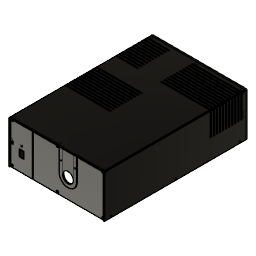
Alt Case (metal) 10mm (Autodesk Fusion 360 design; units mm, degrees)
Autodesk Fusion 360 part; units mm, degrees
sketch "Front" plane through (0, -75, 0) normal (0, -1, 0) x (1, 0, 0)
  line L0 (105, 0) -> (-170, 0)
  line L1 (-170, 0) -> (-170, -10)
  line L2 (-170, -10) -> (107, -10)
  line L3 (-170, 115) -> (105, 115)
  line L4 (-170, 115) -> (-170, 0)
  line L5 (-170, 0) -> (-170, -10)
  line L6 (105, 115) -> (105, 0)
  line L7 (-172, 117) -> (-172, -10)
  line L8 (-172, 117) -> (107, 117)
  line L9 (107, 117) -> (107, -10)
  line L10 (-170, -10) -> (-172, -10)
  circle A0 centre (0, 48) radius 12.5 construction
  line L11 (-104.1, 115) -> (-104.1, -10)
  line L12 (-105.9, 115) -> (-105.9, -10)
  line L13 (-105.9, -10) -> (-104.1, -10)
  line L14 (-144.45, 48) -> (-131.45, 48)
  line L15 (-131.45, 48) -> (-131.45, 28)
  line L16 (-131.45, 28) -> (-144.45, 28)
  line L17 (-144.45, 28) -> (-144.45, 48)
  line L18 (-131.45, 38) -> (-105.9, 38) construction
  line L19 (-144.45, 38) -> (-170, 38) construction
  circle A1 centre (-137.95, 58) radius 1.6
  circle A2 centre (-137.95, 58) radius 3.5
  line L20 (-108, 115) -> (-102, 115)
  line L21 (-102, 115) -> (-102, -10)
  line L22 (-102, -10) -> (-108, -10)
  line L23 (-108, -10) -> (-108, 115)
  line L24 (-105, 115) -> (-105, 111.6183) construction
  line L25 (-105.9, 104.1973) -> (-104.1, 104.1973) construction
  line L26 (-105, 115) -> (-105, -10)
  line L27 (-102, 106) -> (-108, 106)
  line L28 (-15.3704, -10) -> (15.3704, -10)
  line L29 (-12.8704, 115) -> (-17.8704, 115)
  line L30 (105, 115) -> (97, 115)
  line L31 (97, 115) -> (97, 107)
  line L32 (97, 107) -> (105, 107)
  line L33 (105, 107) -> (105, 115)
  line L34 (105, 115) -> (97, 107) construction
  line L35 (97, 115) -> (105, 107) construction
  line L36 (-36.5, 115) -> (-28.5, 115)
  line L37 (-28.5, 115) -> (-28.5, 107)
  line L38 (-28.5, 107) -> (-36.5, 107)
  line L39 (-36.5, 107) -> (-36.5, 115)
  line L40 (-36.5, 115) -> (-28.5, 107) construction
  line L41 (-28.5, 115) -> (-36.5, 107) construction
  line L42 (-170, 115) -> (-162, 115)
  line L43 (-162, 115) -> (-162, 107)
  line L44 (-162, 107) -> (-170, 107)
  line L45 (-170, 107) -> (-170, 115)
  line L46 (-170, 115) -> (-162, 107) construction
  line L47 (-162, 115) -> (-170, 107) construction
  line L48 (105, 57.5) -> (97, 57.5)
  line L49 (97, 57.5) -> (97, 49.5)
  line L50 (97, 49.5) -> (105, 49.5)
  line L51 (105, 49.5) -> (105, 57.5)
  line L52 (105, 57.5) -> (97, 49.5) construction
  line L53 (97, 57.5) -> (105, 49.5) construction
  line L54 (-170, 57.5) -> (-162, 57.5)
  line L55 (-162, 57.5) -> (-162, 49.5)
  line L56 (-162, 49.5) -> (-170, 49.5)
  line L57 (-170, 49.5) -> (-170, 57.5)
  line L58 (-170, 57.5) -> (-162, 49.5) construction
  line L59 (-162, 57.5) -> (-170, 49.5) construction
  line L60 (-200, 53.5) -> (146.6101, 53.5) construction
  circle A3 centre (-32.5, 111) radius 1.45
  circle A4 centre (101, 111) radius 1.45
  circle A5 centre (101, 53.5) radius 1.45
  circle A6 centre (-166, 111) radius 1.45
  circle A7 centre (-166, 53.5) radius 1.45
  line L61 (-28.5, 107) -> (-20.5, 115)
  line L62 (-28.5, 107) -> (-32.5, 107) construction
  line L63 (-85.5, -10) -> (-124.5, -10)
  line L64 (-124.5, -10) -> (-124.5, 20)
  line L65 (-124.5, 20) -> (-85.5, 20)
  line L66 (-85.5, 20) -> (-85.5, -10)
  line L67 (-85.5, -10) -> (-124.5, 20) construction
  line L68 (-124.5, -10) -> (-85.5, 20) construction
  line L69 (61.5, -10) -> (22.5, -10)
  line L70 (22.5, -10) -> (22.5, 20)
  line L71 (22.5, 20) -> (61.5, 20)
  line L72 (61.5, 20) -> (61.5, -10)
  line L73 (61.5, -10) -> (22.5, 20) construction
  line L74 (22.5, -10) -> (61.5, 20) construction
  line L75 (97, 57.5) -> (105, 65.5)
  line L76 (97, 57.5) -> (106.5359, 57.5) construction
  line L77 (105, 0) -> (105, -10)
  line L78 (15.5, 48) -> (15.5, 115)
  line L79 (-15.5, 115) -> (-15.5, 48)
  line L80 (-162, 57.5) -> (-170, 65.5)
  line L81 (-162, 57.5) -> (-152.8212, 57.5) construction
  line L82 (12.5, 0) -> (2.5, 0)
  line L83 (2.5, 0) -> (2.5, 5)
  line L84 (2.5, 5) -> (12.5, 5)
  line L85 (12.5, 5) -> (12.5, 0)
  line L86 (-155, 0) -> (-145, 0)
  line L87 (-145, 0) -> (-145, 5)
  line L88 (-145, 5) -> (-155, 5)
  line L89 (-155, 5) -> (-155, 0)
  circle A8 centre (-166, -5) radius 1.75
  circle A9 centre (-32.5, -5) radius 1.75
  circle A10 centre (101, -5) radius 1.75
  arc A11 (-15.5, 48) -> (15.5, 48) centre (0, 48) ccw
  line L90 (-25.5, 115) -> (-25.5, 48)
  arc A12 (-25.5, 48) -> (25.5, 48) centre (0, 48) ccw
  line L91 (25.5, 48) -> (25.5, 115)
  circle A13 centre (0, 48) radius 15.5
  circle A14 centre (20.5, 81.5) radius 1.75
  circle A15 centre (-20.5, 81.5) radius 1.75
  line L92 (-25.5, 81.5) -> (-15.5, 81.5) construction
  line L93 (15.5, 81.5) -> (25.5, 81.5) construction
  line L94 (0, 48) -> (0, 115) construction
  point P0 (-137.95, 48)
  point P1 (-105, 104.1973)
  point P2 (101, 111)
  point P3 (-32.5, 111)
  point P4 (-166, 111)
  point P5 (101, 53.5)
  point P6 (-166, 53.5)
  point P7 (-105, 5)
  point P8 (42, 5)
  point P9 (-32.5, 117)
  point P10 (0, 81.5)
  dimension "d597" = 2
  dimension "d607" = 115
  dimension "d617" = 105
  dimension "d623" = 1.8
  dimension "d625" = 13
  dimension "d626" = 20
  dimension "d628" = 3.2
  dimension "d629" = 7
  dimension "d630" = 10
  dimension "d634" = 6
  dimension "d639" = 9
  dimension "d806" = 8
  dimension "d808" = 2.9
  dimension "d812" = 45
  dimension "d841" = 39
  dimension "d842" = 30
  dimension "d846" = 65
  dimension "d847" = 65
  dimension "d870" = 45
  dimension "d1" = 275
  dimension "d2" = 48
  dimension "d3" = 25
  dimension "d4" = 31
  dimension "d6" = 53.5
  dimension "d24" = 10
  dimension "d30" = 135
  dimension "d49" = 10
  dimension "d50" = 5
  dimension "d51" = 10
  dimension "d52" = 15
  dimension "d95" = 3.5
  dimension "d97" = 5
  dimension "d100" = 267
  dimension "d101" = 0
  dimension "d102" = 10
  dimension "d103" = 3.5
  dimension "d111" = 4
  constraint horizontal L3
  constraint coincident L0.end L1.start
  constraint coincident L1.end L2.start
  constraint coincident L0.start L6.end
  constraint coincident L3 L11.start
  constraint coincident L2 L11.end
  constraint perpendicular L2 L11
  constraint perpendicular L11 L13
  constraint horizontal L14
  constraint vertical L15
  constraint horizontal L16
  constraint vertical L17
  constraint midpoint L15 L18.start
  constraint coincident L12 L18.end
  constraint perpendicular L12 L18
  constraint midpoint L17 L19.start
  constraint coincident L4 L19.end
  constraint perpendicular L17 L19
  constraint equal L18 L19
  constraint concentric A1 A2
  constraint midpoint L14 P0
  constraint vertical A1.centre P0
  constraint horizontal L20
  constraint vertical L21
  constraint horizontal L22
  constraint vertical L23
  constraint coincident L2 L21.end
  constraint midpoint L20 L24.start
  constraint perpendicular L20 L24
  constraint coincident L12 L25.start
  constraint coincident L11 L25.end
  constraint perpendicular L11 L25
  constraint midpoint L25 P1
  constraint vertical L24.end P1
  constraint coincident L3 L20.start
  constraint midpoint L22 L26.end
  constraint coincident L21 L27.start
  constraint coincident L23 L27.end
  constraint perpendicular L23 L27
  constraint horizontal A0.centre P0
  constraint coincident L2 L28.start
  constraint coincident L2 L28.end
  constraint perpendicular L3 L4
  constraint perpendicular L3 L6
  constraint horizontal L30
  constraint perpendicular L30 L31
  constraint parallel L30 L32
  constraint parallel L31 L33
  constraint coincident L34 P2
  constraint coincident L35 P2
  constraint horizontal L36
  constraint perpendicular L36 L37
  constraint parallel L36 L38
  constraint parallel L37 L39
  constraint coincident L40 P3
  constraint coincident L41 P3
  constraint coincident L3 L36.start
  constraint horizontal L42
  constraint perpendicular L42 L43
  constraint parallel L42 L44
  constraint parallel L43 L45
  constraint coincident L46 P4
  constraint coincident L47 P4
  constraint horizontal L48
  constraint perpendicular L48 L49
  constraint parallel L48 L50
  constraint parallel L49 L51
  constraint coincident L52 P5
  constraint coincident L53 P5
  constraint coincident L6 L48.start
  constraint horizontal L54
  constraint perpendicular L54 L55
  constraint parallel L54 L56
  constraint parallel L55 L57
  constraint coincident L58 P6
  constraint coincident L59 P6
  constraint coincident L4 L54.start
  constraint vertical L31.end L48.end
  constraint vertical L43.end L54.end
  constraint horizontal L31.end L37.end
  constraint horizontal L31.end L43.end
  constraint perpendicular L21 L60
  constraint coincident P6 L60
  constraint coincident P5 L60
  constraint coincident P3 A3.centre
  constraint equal L38 L39
  constraint equal L32 L38
  constraint equal L31 L49
  constraint equal L39 L55
  constraint equal L38 L44
  constraint coincident P2 A4.centre
  constraint coincident P5 A5.centre
  constraint coincident P4 A6.centre
  constraint coincident P6 A7.centre
  constraint equal A3 A4
  constraint equal A3 A7
  constraint equal A3 A5
  constraint equal A3 A6
  constraint horizontal L62
  constraint coincident L3 L61.end
  constraint horizontal L63
  constraint perpendicular L63 L64
  constraint parallel L63 L65
  constraint parallel L64 L66
  constraint coincident L67 P7
  constraint coincident L68 P7
  constraint coincident L26 P7
  constraint coincident L2 L63.start
  constraint horizontal L69
  constraint perpendicular L69 L70
  constraint parallel L69 L71
  constraint parallel L70 L72
  constraint coincident L73 P8
  constraint coincident L74 P8
  constraint coincident L2 L69.start
  constraint equal L66 L72
  constraint equal L65 L71
  constraint horizontal L76
  constraint coincident L6 L75.end
  constraint vertical L12
  constraint vertical origin A0.centre
  constraint coincident A0.centre A11.centre
  constraint coincident origin L0
  constraint coincident L3 L12.start
  constraint coincident L3 L29.end
  constraint coincident L2.end L9.end
  constraint coincident L2 L77.end
  constraint perpendicular L2 L77
  constraint perpendicular L7 L10
  constraint perpendicular L5 L10
  constraint horizontal L78.start L79.end
  constraint tangent L79 A11
  constraint tangent L78 A11
  constraint vertical P3 L62.end
  constraint midpoint L8 P9
  constraint vertical P3 P9
  constraint horizontal L81
  constraint coincident L4 L80.end
  constraint horizontal L82
  constraint vertical L83
  constraint horizontal L84
  constraint vertical L85
  constraint coincident L0 L82.start
  constraint horizontal L86
  constraint vertical L87
  constraint horizontal L88
  constraint vertical L89
  constraint coincident L0 L86.start
  constraint equal L84 L88
  constraint equal L85 L87
  constraint coincident L3 L78.end
  constraint coincident L3 L79.start
  constraint perpendicular L3 L78
  constraint perpendicular L3 L79
  constraint concentric A0 A13
  constraint coincident L78.start A13
  constraint equal A14 A15
  constraint coincident L90 L92.start
  constraint coincident L79 L92.end
  constraint perpendicular L79 L92
  constraint midpoint A15.centre L92
  constraint coincident L78 L93.start
  constraint coincident L91 L93.end
  constraint perpendicular L91 L93
  constraint horizontal L92.end L93.start
  constraint midpoint A14.centre L93
  constraint coincident L3 L94.end
  constraint perpendicular L3 L94
  constraint midpoint L94 P10
  constraint horizontal A14.centre P10
  constraint vertical P6 A8.centre
  measures "d607" distance of L0 L3
  measures "d617" horizontal distance of L0.start A0.centre
  measures "d625" distance of L14.start L14.end
  measures "d626" distance of L14.start L16.end
  measures "d628" diameter of A1
  measures "d629" diameter of A2
  measures "d630" distance of L14 A1.centre
  measures "d634" distance of L21 L23
  measures "d639" distance of L3 L27
  measures "d806" distance of L36.start L38.end
  measures "d808" diameter of A3
  measures "d812" angle of L61 L62
  measures "d841" distance of L64.end L65.end
  measures "d842" distance of L63.end L64.end
  measures "d846" distance of L1.end L26.end
  measures "d847" horizontal distance of L2.end P8
  measures "d870" angle of L75 L76
  measures "d1" distance of L0.end L0.start
  measures "d2" vertical distance of L0.start A0.centre
  measures "d3" diameter of A0
  measures "d4" diameter of A11
  measures "d6" vertical distance of L0.end L60.start
  measures "d24" vertical distance of L0.start L2.end
  measures "d30" angle of L80 L81
  measures "d49" distance of L83.end L84.end
  measures "d50" distance of L82.end L83.end
  measures "d51" distance of L70 L84.end
  measures "d52" distance of L4 L88.end
  measures "d95" diameter of A8
  measures "d97" vertical distance of origin A8.centre
  measures "d103" diameter of A14
  measures "d111" horizontal distance of L0.end A8.centre
extrude "Extrude1" add sketch "Front" along normal blind 1.8 contours L0 L2 L28 L66 L70 L82 | L0 L3 L6 L21 L31 L32 L38 L39 L49 L50 L61 L65 L66 L70 L71 L72 L75 L83 L84 L85 L90 A12 L91 | L0 L82 L83 L84 L85 | L0 L70 L71 L72 | L0 L2 L69 L70 L72 | L0 L2 L21 L63 L66 | L0 L21 L65 L66 | L0 L2 L72 L77 | L0 L2 L11 L21 L22 L63 | L0 L11 L21 L65 | L0 L2 L11 L13 L22 L26 L63 | L0 L11 L26 L65 | L11 L21 L27 L65 | L6 L48 L49 L50 L51 | L0 L2 L12 L13 L22 L26 L63 | L0 L12 L26 L65 | L11 L26 L27 L65 | L3 L11 L20 L21 L27 | L6 L48 L75 | L0 L2 L12 L22 L23 L63 | L0 L12 L23 L65 | L12 L26 L27 L65 | L3 L11 L20 L26 L27 | L0 L2 L23 L63 L64 | L0 L23 L64 L65 | L12 L23 L27 L65 | L3 L12 L20 L26 L27 | L3 L36 L37 L38 L39 | L3 L6 L30 L31 L32 L33 | L0 L1 L2 L5 L64 L86 | L0 L3 L4 L23 L43 L44 L55 L56 L64 L65 L80 L87 L88 L89 | L3 L12 L20 L23 L27 | L3 L37 L61 L90 | L0 L86 L87 L88 L89 | L3 L61 L90 | L3 L29 L61 L78 L79 A11 L90 A12 L91 A13 | L3 L4 L42 L43 L44 L45 | L3 L29 L78 L79 A13 | L4 L54 L55 L56 L57 | A11 A13 | L4 L54 L80 | L14 L15 L16 L17 | A1 | A2 | A3 | A4 | A5 | A6 | A7 | A14 | A15 makes body 1
extrude "Extrude6" cut sketch "Front" against normal blind 0.4 from surface at 1.8 contours L0 L2 L11 L13 L22 L26 L63 | L0 L11 L26 L65 | L0 L2 L12 L13 L22 L26 L63 | L0 L12 L26 L65 | L11 L26 L27 L65 | L12 L26 L27 L65 | L3 L11 L20 L26 L27 | L3 L12 L20 L26 L27 bodies 1
extrude "Extrude2" add sketch "Front" along normal blind 5 and the other way blind 415 separate body contours L1 L2 L3 L4 L5 L6 L7 L8 L9 L10 L20 L29 L30 L33 L36 L42 L45 L51 L57 L77 makes body 2
ref_plane "WorkPlane1" through (-32.5, 130, 53.5) normal (0, -1, 0) x (0, 0, -1)
mirror "Mirror2" about plane through (-32.5, 130, 53.5) normal (0, -1, 0) of bodies 1 makes body 3
extrude "Extrude41" add sketch "Front" against normal blind 1.2 contours A2 bodies 1
extrude "Extrude42" cut sketch "Front" along normal through all contours L3 L29 L78 L79 A13 | A11 A13 | L14 L15 L16 L17 | A1 bodies 1
sketch "cutouts rear" plane through (0, 336.8, 0) normal (0, 1, 0) x (-1, 0, 0)
  line L0 (105.9, -18) -> (170, -18)
  line L1 (170, 110) -> (105.9, 110)
  circle A0 centre (65, 10) radius 3.75
  line L2 (170, -18) -> (-105, -18)
  line L3 (130.5, 36.5) -> (144.5, 36.5)
  line L4 (144.5, 36.5) -> (144.5, 27.5)
  line L5 (144.5, 27.5) -> (130.5, 27.5)
  line L6 (130.5, 27.5) -> (130.5, 36.5)
  circle A1 centre (151.25, 32) radius 1.6
  circle A2 centre (123.75, 32) radius 1.6
  line L7 (123.75, 32) -> (151.25, 32) construction
  line L8 (105.9, 110) -> (105.9, -18)
  line L9 (170, -18) -> (170, 110)
  line L10 (104.1, -10) -> (104.1, 115)
  line L11 (-105, -10) -> (104.1, -10)
  line L12 (105, -18) -> (105, 115)
  circle A3 centre (130, 17) radius 3.5
  circle A4 centre (145, 17) radius 3.5
  line L13 (104.1, 115) -> (-105, 115)
  line L14 (-105, 115) -> (-105, -10)
  line L15 (104.1, 115) -> (-105, 115)
  line L16 (-105, 115) -> (-105, -10)
  line L17 (-105, -10) -> (104.1, -10)
  line L18 (130, 17) -> (145, 17) construction
  circle A5 centre (-101, -5) radius 1.75
  circle A6 centre (32.5, -5) radius 1.75
  line L19 (104.1, -10) -> (104.1, 115)
  circle A7 centre (-101, 53.5) radius 1.45
  circle A8 centre (-101, 111) radius 1.45
  circle A9 centre (32.5, 111) radius 1.45
  circle A10 centre (166, 111) radius 1.45
  circle A11 centre (166, 53.5) radius 1.45
  circle A12 centre (166, -5) radius 1.75
  circle A13 centre (32.5, -5) radius 1.75
  circle A14 centre (-101, -5) radius 1.75
  point P0 (170, 0)
  point P1 (144.5, 32)
  point P2 (137.5, 32)
  point P3 (137.5, 36.5)
  point P4 (137.5, 17)
  point P5 (-101, 111)
  point P6 (32.5, 111)
  point P7 (-101, 53.5)
  point P8 (166, 111)
  point P9 (166, 53.5)
  dimension "d675" = 7.5
  dimension "d678" = 9
  dimension "d679" = 14
  dimension "d680" = 3.2
  dimension "d681" = 27.5
  dimension "d683" = 50
  dimension "d849" = 18.75
  dimension "d851" = 10
  dimension "d853" = 40
  dimension "d854" = 18.75
  dimension "d868" = 7
  dimension "d871" = 35
  dimension "d19" = 15
  dimension "d92" = 15
  constraint horizontal L3
  constraint vertical L4
  constraint horizontal L5
  constraint vertical L6
  constraint equal A1 A2
  constraint midpoint L4 P1
  constraint horizontal A1.centre P1
  constraint horizontal A1.centre A2.centre
  constraint coincident A2.centre L7.start
  constraint coincident A1.centre L7.end
  constraint midpoint L7 P2
  constraint midpoint L3 P3
  constraint vertical P2 P3
  constraint equal A3 A4
  constraint horizontal A3.centre A4.centre
  constraint coincident A3.centre L18.start
  constraint coincident A4.centre L18.end
  constraint midpoint L18 P4
  constraint vertical P2 P4
  measures "d675" diameter of A0
  measures "d678" distance of L3.start L5.end
  measures "d679" distance of L3.start L3.end
  measures "d680" diameter of A1
  measures "d681" distance of A1.centre A2.centre
  measures "d683" distance of L0 P2
  measures "d849" distance of A1.centre L9
  measures "d851" vertical distance of origin A0.centre
  measures "d853" distance of A0.centre L12
  measures "d854" distance of A2.centre L12
  measures "d868" diameter of A3
  measures "d871" distance of L2 A3.centre
  measures "d19" distance of A3.centre A4.centre
  measures "d92" distance of P2 P4
extrude "Cable cutouts" cut sketch "cutouts rear" against normal up to surface (1.8 mm away) contours L1 A10 | A0 | L3 L4 L5 L6 | A1 | A2 | A3 | A4 | A7 | A8 | A9 | A11 picked at (166.4266, 111.329) bodies 3
sketch "Grille" plane through (-170, 0, 0) normal (1, 0, 0) x (0, 1, 0)
  line L0 (328, 104.1341) -> (-78, 104.1341)
  line L1 (-78, 104.1341) -> (-78, -5.9329)
  line L2 (-78, -5.9329) -> (328, -5.9329)
  line L3 (328, -5.9329) -> (328, 104.1341)
  line L4 (325, 104.0001) -> (325, -23.9219)
  line L5 (-78, 104.1341) -> (328, 104.1341)
  circle A0 centre (269.25, 65.3841) radius 40
  line L6 (305, 29.6341) -> (233.5, 29.6341)
  line L7 (233.5, 29.6341) -> (233.5, 101.1341)
  line L8 (233.5, 101.1341) -> (305, 101.1341)
  line L9 (305, 101.1341) -> (305, 29.6341)
  line L10 (305, 29.6341) -> (233.5, 101.1341) construction
  line L11 (233.5, 29.6341) -> (305, 101.1341) construction
  circle A1 centre (233.5, 101.1341) radius 2.5
  circle A2 centre (305, 101.1341) radius 2.5
  circle A3 centre (305, 29.6341) radius 2.5
  circle A4 centre (233.5, 29.6341) radius 2.5
  circle A5 centre (269.25, 65.3841) radius 32.5
  circle A6 centre (269.25, 65.3841) radius 25
  circle A7 centre (269.25, 65.3841) radius 17.5
  circle A8 centre (269.25, 65.3841) radius 10
  circle A9 centre (269.25, 65.3841) radius 5
  circle A10 centre (269.25, 65.3841) radius 34.5
  circle A11 centre (269.25, 65.3841) radius 27
  circle A12 centre (269.25, 65.3841) radius 19.5
  circle A13 centre (269.25, 65.3841) radius 12
  line L12 (234.9142, 28.2199) -> (306.4142, 99.7199)
  line L13 (232.0858, 31.0483) -> (303.5858, 102.5483)
  line L14 (306.4142, 31.0483) -> (234.9142, 102.5483)
  line L15 (303.5858, 28.2199) -> (232.0858, 99.7199)
  line L16 (328, -18) -> (-78, -18)
  line L17 (-78, -18) -> (-78, 112)
  line L18 (-78, 112) -> (328, 112)
  line L19 (328, 112) -> (328, -18)
  line L20 (340, 115) -> (-80, 115)
  line L21 (-80, 115) -> (-80, -10)
  line L22 (-80, -10) -> (340, -10)
  line L23 (340, -10) -> (340, 115)
  point P0 (269.25, 65.3841)
  dimension "d690" = 80
  dimension "d691" = 71.5
  dimension "d692" = 71.5
  dimension "d693" = 5
  dimension "d694" = 3
  dimension "d695" = 20
  dimension "d696" = 65
  dimension "d697" = 50
  dimension "d698" = 35
  dimension "d699" = 20
  dimension "d700" = 10
  dimension "d701" = 2
  dimension "d702" = 2
  dimension "d703" = 2
  dimension "d704" = 2
  dimension "d705" = 2
  dimension "d706" = -2
  dimension "d707" = 2
  dimension "d708" = -2
  constraint horizontal L6
  constraint perpendicular L6 L7
  constraint parallel L6 L8
  constraint parallel L7 L9
  constraint coincident L10 P0
  constraint coincident L11 P0
  constraint coincident P0 A0.centre
  constraint coincident L7.end L8.start
  constraint coincident L8.end L9.start
  constraint coincident L6.start L9.end
  constraint coincident L6.end L7.start
  constraint equal A1 A2
  constraint equal A1 A4
  constraint equal A1 A3
  constraint concentric A0 A5
  constraint concentric A0 A6
  constraint concentric A5 A7
  constraint concentric A5 A8
  measures "d690" diameter of A0
  measures "d691" distance of L7.end L8.end
  measures "d692" distance of L6.end L7.end
  measures "d693" diameter of A1
  measures "d694" distance of L5 L8
  measures "d695" distance of L4 L9
  measures "d696" diameter of A5
  measures "d697" diameter of A6
  measures "d698" diameter of A7
  measures "d699" diameter of A8
  measures "d700" diameter of A9
sketch "Cooling slots" plane through (0, 0, 117) normal (0, 0, 1) x (-1, 0, 0)
  line L0 (172, 80) -> (-107, 80)
  line L1 (38, -322) -> (38, -325)
  line L2 (38, -322) -> (-107, -325) construction
  line L3 (38, -325) -> (-107, -325)
  line L4 (-107, -322) -> (38, -325) construction
  line L5 (-107, -322) -> (38, -322)
  line L6 (-36, -322) -> (-33, -322)
  line L7 (-33, -322) -> (-33, -325)
  line L8 (-33, -325) -> (-36, -325)
  line L9 (-36, -325) -> (-36, -322)
  line L10 (-36, -322) -> (-33, -325) construction
  line L11 (-33, -322) -> (-36, -325) construction
  line L12 (-107, 80) -> (-107, -340)
  line L13 (182.5619, -325) -> (106.329, -325)
  line L14 (106.329, -325) -> (106.329, -322)
  line L15 (106.329, -322) -> (182.5619, -322)
  line L16 (182.5619, -322) -> (182.5619, -325)
  line L17 (182.5619, -325) -> (106.329, -322) construction
  line L18 (106.329, -325) -> (182.5619, -322) construction
  line L19 (-107, -322) -> (-107, -325)
  line L20 (189.5022, -173) -> (189.5022, -176)
  line L21 (106.329, -173) -> (106.329, -176)
  line L22 (106.329, -173) -> (189.5022, -176) construction
  line L23 (189.5022, -176) -> (106.329, -176)
  line L24 (103.329, -176) -> (38, -176)
  line L25 (38, -176) -> (103.329, -173) construction
  line L26 (106.329, -173) -> (189.5022, -173)
  line L27 (189.5022, -173) -> (106.329, -176) construction
  line L28 (103.329, -173) -> (103.329, -176)
  line L29 (38, -173) -> (103.329, -173)
  line L30 (38, -176) -> (38, -173)
  line L31 (103.329, -176) -> (38, -173) construction
  line L32 (-107, -130) -> (10, -130)
  line L33 (172, -340) -> (172, 80)
  line L34 (105, 75) -> (104.7222, -328) construction
  line L35 (-107, -340) -> (172, -340)
  point P0 (-34.5, -323.5)
  point P1 (-34.5, -323.5)
  point P2 (144.4455, -323.5)
  point P3 (147.9156, -174.5)
  point P4 (70.6645, -174.5)
  point P5 (105, 75)
  dimension "d727" = 3
  dimension "d730" = 145
  dimension "d813" = 3
  dimension "d32" = 15
  dimension "d35" = 3
  dimension "d38" = 43
  dimension "d71" = 1.5
  dimension "d72" = 1.5
  constraint horizontal L5
  constraint perpendicular L1 L5
  constraint parallel L3 L5
  constraint coincident P1 L4
  constraint coincident P1 L2
  constraint horizontal L6
  constraint perpendicular L6 L7
  constraint parallel L6 L8
  constraint parallel L7 L9
  constraint coincident L10 P1
  constraint coincident L11 P1
  constraint coincident P1 P0
  constraint coincident L3 L8.end
  constraint horizontal L13
  constraint perpendicular L13 L14
  constraint parallel L13 L15
  constraint parallel L14 L16
  constraint coincident L17 P2
  constraint coincident L18 P2
  constraint horizontal P1 P2
  constraint horizontal L1.start L14.end
  constraint perpendicular L5 L19
  constraint coincident L4.start L12
  constraint horizontal L26
  constraint perpendicular L20 L26
  constraint parallel L23 L26
  constraint coincident P3 L22
  constraint coincident P3 L27
  constraint coincident L21.end L27
  constraint coincident L21.start L22.start
  constraint coincident L21.end L23.end
  constraint perpendicular L21 L26
  constraint horizontal L24
  constraint perpendicular L24 L30
  constraint parallel L24 L29
  constraint parallel L28 L30
  constraint coincident P4 L31
  constraint coincident P4 L25
  constraint horizontal P3 P4
  constraint horizontal L21.start L25.end
  constraint midpoint L12 L32.start
  constraint perpendicular L12 L32
  constraint coincident P5 L34.start
  constraint vertical L14.end L21.end
  constraint vertical L1.start L24.end
  measures "d727" distance of L1.start L1.end
  measures "d730" distance of L4.start L1.start
  measures "d813" distance of L7.end L8.end
  measures "d32" vertical distance of L12.end L2.end
  measures "d35" distance of L20.start L20.end
  measures "d38" vertical distance of L29.start L32.end
  measures "d71" distance of L21.start L34
  measures "d72" distance of L25.end L34
extrude "Extrude39" cut sketch "Cooling slots" against normal blind 70 contours L3 L5 L9 L12 L19 | L13 L14 L15 L33 | L13 L15 L16 L33 | L1 L3 L5 L7 bodies 2
pattern_linear "R-Pattern1" count 11 spacing 9 along (0, -1, 0) of "Extrude39"
extrude "Extrude40" cut sketch "Cooling slots" against normal blind 70 contours L21 L23 L26 L33 | L20 L23 L26 L33 | L24 L28 L29 L30 bodies 2
pattern_linear "R-Pattern3" count 11 spacing 9 along (0, -1, 0) of "Extrude40"
extrude "Extrude28" add sketch "Front" against normal blind 6 contours L3 L36 L37 L38 L39 | L3 L6 L30 L31 L32 L33 | L3 L4 L42 L43 L44 L45 | L4 L54 L55 L56 L57 | L4 L54 L80 bodies 2
extrude "Extrude29" add sketch "Front" along normal blind 6 from surface at -410 contours L6 L48 L49 L50 L51 | L6 L48 L75 | L3 L36 L37 L38 L39 | L3 L6 L30 L31 L32 L33 | L3 L4 L42 L43 L44 L45 | L4 L54 L55 L56 L57 | L4 L54 L80 bodies 2
sketch "hole guide" plane through (0, -76.8, 0) normal (0, -1, 0) x (1, 0, 0)
  line L0 (105, 110) -> (-104.1, 110)
  line L1 (-170, -10) -> (-170, 115)
  circle A0 centre (-32.5, 111) radius 1.45
  circle A1 centre (101, 111) radius 1.45
  circle A2 centre (-166, 53.5) radius 1.45
  line L2 (105, -10) -> (105, 115)
  line L3 (-15.5, 115) -> (-104.1, 115)
  circle A3 centre (101, -5) radius 1.75
  circle A4 centre (-32.5, -5) radius 1.75
  line L4 (-15.5, 48) -> (-15.5, 115)
  line L5 (105, 115) -> (15.5, 115)
  line L6 (15.5, 115) -> (15.5, 48)
  arc A5 (-15.5, 48) -> (15.5, 48) centre (0, 48) ccw
  circle A6 centre (-166, -5) radius 1.75
  point P0 (0, 106)
  point P1 (101, 106)
  point P2 (-166, 111)
hole "Hole1" at (-166, -76.8, 111) at (-32.5, -76.8, 111) at (101, -76.8, 111) at (-166, -76.8, 53.5) at (-166, -76.8, -5) at (-32.5, -76.8, -5) at (101, -76.8, -5) direction (0, 1, 0) diameter 3.2 depth 3 tip angle 180 countersink diameter 7 countersink angle 90 bodies 1
hole "Hole3" at (101, 336.8, 111) at (-32.5, 336.8, 111) at (-166, 336.8, 111) at (-166, 336.8, 53.5) at (-166, 336.8, -5) at (-32.5, 336.8, -5) at (101, 336.8, -5) at (101, 336.8, 53.5) direction (0, -1, 0) diameter 3.2 depth 3 tip angle 180 countersink diameter 7 countersink angle 90 bodies 2 3
sketch "hole guide side" plane through (107, 0, 0) normal (1, 0, 0) x (0, 1, 0)
  circle A0 centre (-58.8, -5) radius 1.75
  line L0 (232, 117) -> (-80, 117)
  line L1 (322, 117) -> (316, 117)
  line L2 (313, 117) -> (307, 117)
  line L3 (304, 117) -> (298, 117)
  line L4 (295, 117) -> (289, 117)
  line L5 (286, 117) -> (280, 117)
  line L6 (277, 117) -> (271, 117)
  line L7 (268, 117) -> (262, 117)
  line L8 (259, 117) -> (253, 117)
  line L9 (250, 117) -> (244, 117)
  line L10 (241, 117) -> (235, 117)
  line L11 (336.8, 115) -> (336.8, -10)
  line L12 (335, 115) -> (336.8, 115)
  line L13 (335, -10) -> (336.8, -10)
  line L14 (-75, -10) -> (-75, 54.5)
  line L15 (-75, 61.5) -> (-75, 115)
  line L16 (-76.8, 115) -> (-76.8, -10)
  line L17 (-75, 115) -> (-76.8, 115)
  line L18 (-75, -10) -> (-76.8, -10)
  circle A1 centre (130, -5) radius 1.75
  circle A2 centre (318.8, -5) radius 1.75
  line L19 (335, -10) -> (335, 115)
  line L20 (-73.8, 58) -> (-73.8, 61.5)
  line L21 (-73.8, 54.5) -> (-73.8, 58)
  line L22 (-75, 54.5) -> (-73.8, 54.5)
  line L23 (-75, 61.5) -> (-73.8, 61.5)
  line L24 (340, -10) -> (340, 117)
  line L25 (340, 117) -> (325, 117)
  line L26 (-58.8, -5) -> (318.8, -5) construction
  dimension "d839" = 3.5
  dimension "d80" = 18
  dimension "d87" = 5
  dimension "d117" = 18
  constraint horizontal A0.centre A1.centre
  constraint horizontal A0.centre A2.centre
  constraint equal A0 A1
  constraint equal A0 A2
  constraint coincident A0.centre L26.start
  constraint coincident A2.centre L26.end
  constraint midpoint A1.centre L26
  measures "d839" diameter of A0
  measures "d80" distance of A0.centre L16
  measures "d87" vertical distance of origin A0.centre
  measures "d117" distance of L11 A2.centre
extrude "Extrude31" cut sketch "hole guide side" against normal through all contours A0 | A1 | A2 bodies 2
extrude "Extrude32" [suppressed]
fillet "Fillet1" radius 2 58 edges at (107, 332.5, 117) (107, 121, 117) (107, 319, 117) (107, 292, 117) (107, 274, 117) (107, 310, 117) (107, 283, 117) (107, 301, 117) (107, 265, 117) (107, 247, 117) (107, 76, 117) (107, 256, 117) (107, 238, 117) (-172, 1.5, 117) (-172, 332.5, 117) (-172, 319, 117) (-172, 310, 117) (-172, 301, 117) (-172, 292, 117) (-172, 283, 117) (-172, 274, 117) (-172, 265, 117) (-172, 256, 117) (-172, 247, 117) (-172, 238, 117) (-172, 204, 117) (-172, 170, 117) (-172, 161, 117) (-172, 152, 117) (-172, 143, 117) (-172, 134, 117) (-172, 125, 117) (-172, 116, 117) (-172, 107, 117) (-172, 98, 117) (-172, 89, 117) (-172, 319, 117) (-172, 301, 117) (-172, 161, 117) (-172, 310, 117) (-172, 265, 117) (-172, 247, 117) (-172, 292, 117) (-172, 256, 117) (-172, 283, 117) (-172, 274, 117) (-172, 170, 117) (-172, 89, 117) (-172, 143, 117) (-172, 152, 117) (-172, 204, 117) (-172, 238, 117) (-172, 125, 117) (-172, 107, 117) (-172, 134, 117) (-172, 116, 117) (-172, 98, 117) (-172, 1.5, 117) on bodies 2
extrude "Extrude37" [suppressed]
extrude "Extrude38" [suppressed]
extrude "Extrude43" add sketch "Front" along normal blind 2 from surface at 1.8 separate body contours L3 L61 L90 | L3 L29 L61 L78 L79 A11 L90 A12 L91 A13 | L3 L29 L78 L79 A13 makes body 4
extrude "Extrude44" cut sketch "Front" along normal through all contours A14 | A15 bodies 1
thread "Thread1" "ISO Metric profile 3.0 M3x0.5 M3x0.5 6H" major diameter 3.086 minor diameter 2.529 pitch 0.5 angle 60 modelled right hand crest width 0.1368 on face at (-18.8555, -75.6, 82.0985) crest through (-19.2355, -75.125, 81.5) on face at (22.1445, -75.6, 82.0985) crest through (21.7645, -75.125, 81.5) on bodies 1
equation "d847 = d846"
equation "d6 = d607 / 2 - 4 mm"
equation "d80 = d117"
equation "d100 = 275 mm - ( 4 * 2 ) * 1 mm"
named bodies: "Casing-Front-10mm", "Casing-Cover-10mm", "Casing-Rear-10mm", "Casing-Tube cover-10mm"
